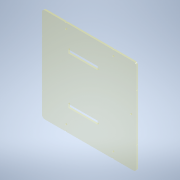
# Autodesk Inventor part: PCB Protector for Small Board
Saved by Autodesk Inventor 2022 (Build 260153000, 153)
## iProperties
Created: 2021-06-21
Part Number: PCB Protector for Small Board
Material: Glass
Document SubType Name: Modeling
Designer: benka
Density: 2.18 g/cm^3
Appearance: Clear - Yellow
Author: benka
Autodesk Inventor part; units mm, degrees
ref_plane "YZ Plane" through (0, 0, 0) normal (1, 0, 0) x (0, 1, 0)
ref_plane "XZ Plane" through (0, 0, 0) normal (0, 1, 0) x (-1, 0, 0)
ref_plane "XY Plane" through (0, 0, 0) normal (0, 0, 1) x (1, 0, 0)
sketch "Sketch1" plane through (-41.0022, 83.9754, 0) normal (0, 0, 1) x (1, 0, 0)
  line L0 (43.6907, -84.1601) -> (79.4807, -84.1601)
  arc A0 (43.6907, -84.1601) -> (41.6657, -84.1611) centre (42.6783, -84.1982) ccw
  line L1 (-40.3343, -84.1601) -> (41.6657, -84.1611)
  arc A1 (-40.3343, -84.1601) -> (-42.3343, -84.1611) centre (-41.3342, -84.1854) ccw
  line L2 (-78.1393, -84.1601) -> (-42.3343, -84.1611)
  arc A2 (-83.3093, -78.9901) -> (-78.1393, -84.1601) centre (-78.1401, -78.9909) ccw
  line L3 (-83.3093, -43.2101) -> (-83.3093, -78.9901)
  arc A3 (-83.3093, -43.2101) -> (-83.3103, -41.1851) centre (-83.3474, -42.1976) ccw
  line L4 (-83.3093, 40.8149) -> (-83.3103, -41.1851)
  arc A4 (-83.3093, 40.8149) -> (-83.3103, 42.8149) centre (-83.3346, 41.8149) ccw
  line L5 (-83.3093, 78.6259) -> (-83.3103, 42.8149)
  arc A5 (-78.1463, 83.7899) -> (-83.3093, 78.6259) centre (-78.147, 78.6276) ccw
  line L6 (-42.3343, 83.7899) -> (-78.1463, 83.7899)
  arc A6 (-42.3343, 83.7899) -> (-40.3343, 83.7899) centre (-41.3343, 83.8153) ccw
  line L7 (41.6657, 83.7899) -> (-40.3343, 83.7899)
  arc A7 (41.6657, 83.7899) -> (43.6657, 83.7909) centre (42.6657, 83.8152) ccw
  line L8 (79.4797, 83.7899) -> (43.6657, 83.7909)
  arc A8 (84.6457, 78.6229) -> (79.4797, 83.7899) centre (79.48, 78.6242) ccw
  line L9 (84.6457, 42.8349) -> (84.6457, 78.6229)
  arc A9 (84.6457, 42.8349) -> (84.6417, 40.8149) centre (84.6762, 41.8249) ccw
  line L10 (84.6407, -41.1851) -> (84.6417, 40.8149)
  arc A10 (84.6407, -41.1851) -> (84.6417, -43.1851) centre (84.666, -42.1851) ccw
  line L11 (84.6407, -79.0001) -> (84.6417, -43.1851)
  arc A11 (79.4807, -84.1601) -> (84.6407, -79.0001) centre (79.4819, -79.0012) ccw
  circle A12 centre (42.6657, 73.3149) radius 1
  circle A13 centre (-41.3343, 73.3149) radius 1
  circle A14 centre (-41.3343, -73.6851) radius 1
  circle A15 centre (42.6657, -73.6851) radius 1
  circle A16 centre (74.1657, -0.1851) radius 1
  line L12 (15.5981, 38.5892) -> (-36.6892, 38.5892)
  line L13 (-36.6892, 38.5892) -> (-36.6892, 44.7944)
  line L14 (-36.6892, 44.7944) -> (15.5981, 44.7944)
  line L15 (15.5981, 44.7944) -> (15.5981, 38.5892)
  line L16 (15.5981, -45.4168) -> (-36.6892, -45.4168)
  line L17 (-36.6892, -45.4168) -> (-36.6892, -39.2116)
  line L18 (-36.6892, -39.2116) -> (15.5981, -39.2116)
  line L19 (15.5981, -39.2116) -> (15.5981, -45.4168)
  point P0 (0.6657, -0.1851)
  point P1 (-10.5892, -42.205)
  point P2 (-10.5892, 41.801)
  point P3 (-10.5892, -42.205)
  constraints: 40 end point, 24 point on circle, 17 centre point, 4 parallel, 2 horizontal, 2 perpendicular
extrude "Extrusion1" add sketch "Sketch1" along normal blind 3
body "Solid1"
